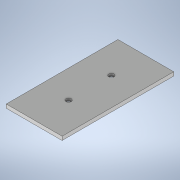
# Autodesk Inventor part: Battery_holder_2
Saved by Autodesk Inventor 2022 (Build 260153000, 153)
## iProperties
Created: 2023-02-02
Part Number: Battery_holder_2
Material: Generic
Document SubType Name: Modeling
Designer: scott
Density: 1 g/cm^3
Appearance: Default
Author: scott
Autodesk Inventor part; units mm, degrees
ref_plane "YZ Plane" through (0, 0, 0) normal (1, 0, 0) x (0, 1, 0)
ref_plane "XZ Plane" through (0, 0, 0) normal (0, 1, 0) x (-1, 0, 0)
ref_plane "XY Plane" through (0, 0, 0) normal (0, 0, 1) x (1, 0, 0)
sketch "Sketch1" plane through (0, 0, 0) normal (0, 1, 0) x (-1, 0, 0)
  line L0 (15, 30) -> (-15, 30)
  line L1 (-15, 30) -> (-15, -30)
  line L2 (-15, -30) -> (15, -30)
  line L3 (15, -30) -> (15, 30)
  line L4 (0, 11.5) -> (-15, 11.5)
  line L5 (-15, 11.5) -> (-15, -11.5)
  line L6 (-15, -11.5) -> (0, -11.5)
  line L7 (0, -11.5) -> (0, 11.5)
  point P0 (0, 0)
  dimension "d0" = 30
  dimension "d1" = 60
  dimension "d2" = 30
  dimension "d3" = 15
  dimension "d4" = 23
  dimension "d5" = 18.5
  constraints: 16 end point, 4 parallel, 2 horizontal, 2 perpendicular, 1 point on line
  measures "d0" distance of L1.end L2.end
  measures "d1" distance of L0.end L1.end
  measures "d2" distance from line of point (0, 0) L2
  measures "d3" distance from line of L1 point (0, 0)
  measures "d4" distance of L6.end L4.start
  measures "d5" distance between parallel lines of L4 L0
extrude "Extrusion1" add sketch "Sketch1" along normal blind 2
hole "Hole1" at (0, 0, -11.5) at (0, 0, 11.5) direction (0, 1, 0) diameter 2.8 end through all counterbore diameter 5 counterbore depth 0.5
equation "\"d2\" = 0.5 * d1"
equation "\"d3\" = 0.5 * d0"
equation "\"d5\" = -0.5 * d4 + 0.5 * d1"
body "Solid1"
